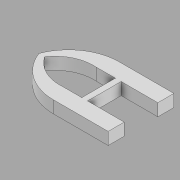
# Autodesk Inventor part: Assignement 1
Saved by Autodesk Inventor 2022 (Build 260153000, 153)
## iProperties
Created: 2021-09-20
Part Number: Assignement 1
Material: Generic
Document SubType Name: Modeling
Designer: seang
Density: 1 g/cm^3
Appearance: Default
Author: seang
Autodesk Inventor part; units mm, degrees
ref_plane "YZ Plane" through (0, 0, 0) normal (1, 0, 0) x (0, 1, 0)
ref_plane "XZ Plane" through (0, 0, 0) normal (0, 1, 0) x (-1, 0, 0)
ref_plane "XY Plane" through (0, 0, 0) normal (0, 0, 1) x (1, 0, 0)
sketch "Sketch2" plane through (0, 0, 0) normal (0, 1, 0) x (-1, 0, 0)
  line L0 (3, -1.3125) -> (3, -4.0625)
  line L1 (3, -4.0625) -> (0, -4.0625)
  line L2 (3.4688, -4.0625) -> (5.0312, -4.0625)
  arc A0 (7.875, -2.6875) -> (5.0312, -1.3125) centre (5.2784, -4.4296) ccw
  arc A1 (5.0312, -4.0625) -> (7.875, -2.6875) centre (5.2784, -0.9454) ccw
  arc A2 (8.3438, -2.6875) -> (4.4576, 0) centre (4.4576, -4.1534) ccw
  arc A3 (4.4576, -5.375) -> (8.3438, -2.6875) centre (4.4576, -1.2216) ccw
  line L3 (4.4576, -5.375) -> (0, -5.375)
  line L4 (3.4688, -1.3125) -> (3.4688, -4.0625)
  line L5 (5.0312, -1.3125) -> (3.4688, -1.3125)
  line L6 (0, -5.375) -> (0, -4.0625)
  line L7 (3, -1.3125) -> (0, -1.3125)
  line L8 (0, -1.3125) -> (0, 0)
  line L9 (4.4576, 0) -> (0, 0)
  dimension "d2" = 1.3125
  dimension "d5" = 1.5625
  dimension "d7" = 0.4688
  dimension "d10" = 3
  dimension "d14" = 4.4576
  dimension "d15" = 2.75
  constraints: 20 end point, 8 equal length, 8 point on circle, 4 centre point, 3 horizontal, 3 perpendicular, 2 equal radius, 1 vertical
  measures "d2" distance of L1.end L3.end
  measures "d5" distance of L2.start L2.end
  measures "d7" distance of A0.start A2.start
  measures "d10" distance of L0.start L7.end
  measures "d14" distance of L3.start L3.end
  measures "d15" distance of L0.start L0.end
extrude "Extrusion2" add sketch "Sketch2" along normal blind 1
body "Solid2"
